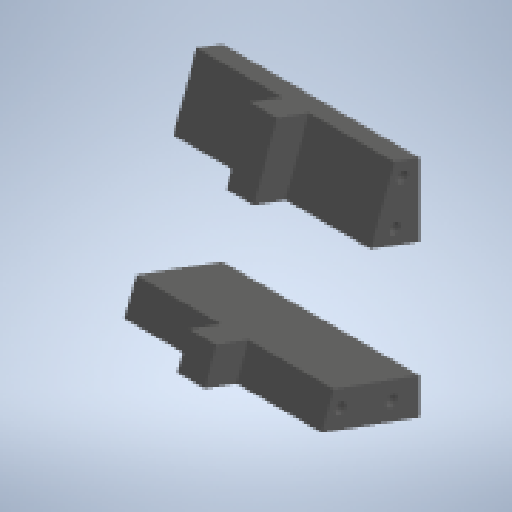
# Autodesk Inventor part: chest_cover_bace
Saved by Autodesk Inventor 2024.1 (Build 281209000, 209)
## iProperties
Created: 2024-02-14
Part Number: chest_cover_bace
Material: 一般
Document SubType Name: Modeling
Designer: hibik
Density: 1 g/cm^3
Appearance: 既定
Author: hibik
Autodesk Inventor part; units mm, degrees
ref_plane "YZ Plane" through (0, 0, 0) normal (1, 0, 0) x (0, 1, 0)
ref_plane "XZ Plane" through (0, 0, 0) normal (0, 1, 0) x (-1, 0, 0)
ref_plane "XY Plane" through (0, 0, 0) normal (0, 0, 1) x (1, 0, 0)
sketch "スケッチ1" plane through (0, 0, 0) normal (1, 0, 0) x (0, 1, 0)
  line L0 (0, 0) -> (33, 0)
  line L1 (33, 0) -> (3.8603, 10.606)
  line L2 (3.8603, 10.606) -> (0, 0)
  line L3 (33, 0) -> (3.8603, 10.606)
  line L4 (3.8603, 10.606) -> (5.2283, 14.3648)
  line L5 (5.2283, 14.3648) -> (34.3681, 3.7588)
  line L6 (34.3681, 3.7588) -> (33, 0)
  dimension "d0" = 33
  dimension "d1" = 20
  dimension "d2" = 4
  constraints: 14 end point, 3 equal length, 2 perpendicular, 1 horizontal
  measures "d0" distance of L0.start L0.end
  measures "d1" angle of L0 L1
  measures "d2" distance between parallel lines of L5 L1
extrude "押し出し1" add sketch "スケッチ1" along normal blind 16.5
sketch "スケッチ2" plane through (0, 5.2283, 14.3648) normal (0, 0.3420201, 0.9396926) x (1, 0, 0)
  line L0 (0, 31.0099) -> (16.5, 31.0099) projected
  line L1 (16.5, 31.0099) -> (16.5, 0) projected
  line L2 (12.5, 31.0099) -> (16.5, 31.0099)
  line L3 (16.5, 31.0099) -> (16.5, 0)
  line L4 (16.5, 0) -> (12.5, 0)
  line L5 (12.5, 0) -> (12.5, 31.0099)
  point P0 (0, 0)
  dimension "d5" = 4
  constraints: 8 end point, 2 parallel, 1 horizontal, 1 perpendicular, 1 point on line
  measures "d5" distance between parallel lines of L1 L5
extrude "押し出し2" add sketch "スケッチ2" along normal blind 5
extrude "押し出し3" add sketch "スケッチ1" along normal blind 29
sketch "スケッチ3" plane through (0, 0, 0) normal (-1, 0, 0) x (0, 0, 1)
  line L0 (3.7588, 34.3681) -> (14.3648, 5.2283) projected
  line L1 (7.179, 24.9712) -> (12.6547, 9.9268)
  line L2 (12.6547, 9.9268) -> (0, 5.3209)
  line L3 (0, 5.3209) -> (-5.4757, 20.3652)
  line L4 (-5.4757, 20.3652) -> (7.179, 24.9712)
  line L5 (0, 0) -> (0, 33) projected
  line L6 (0, 33) -> (3.7588, 34.3681) projected
  line L7 (14.3648, 5.2283) -> (0, 0) projected
  circle A0 centre (11.6303, 6.8935) radius 0.8
  circle A1 centre (4.1128, 4.1574) radius 0.8
  circle A2 centre (2.5634, 31.8047) radius 0.8
  circle A3 centre (3.6759, 25.8245) radius 0.8
  line L8 (7.179, 24.9712) -> (12.6547, 9.9268)
  line L9 (12.6547, 9.9268) -> (17.3531, 11.6369)
  line L10 (17.3531, 11.6369) -> (11.8774, 26.6813)
  line L11 (11.8774, 26.6813) -> (7.179, 24.9712)
  point P0 (0, 22.3582)
  dimension "d13" = 10
  dimension "d14" = 5
  dimension "d15" = 1.6
  dimension "d16" = 1.6
  dimension "d17" = 1.6
  dimension "d18" = 1.6
  dimension "d19" = 2.5
  dimension "d20" = 2.5
  dimension "d21" = 2
  dimension "d22" = 3
  dimension "d23" = 2
  dimension "d24" = 2
  dimension "d25" = 2
  dimension "d26" = 10
  constraints: 16 end point, 4 centre point, 4 parallel, 3 point on line, 2 perpendicular, 1 collinear
  measures "d13" distance between parallel lines of L6 L4
  measures "d14" distance between parallel lines of L7 L2
  measures "d15" diameter of A0
  measures "d16" diameter of A1
  measures "d17" diameter of A2
  measures "d18" diameter of A3
  measures "d19" distance from line of L7 A0.centre
  measures "d20" distance from line of L7 A1.centre
  measures "d21" distance from line of L0 A2.centre
  measures "d22" distance from line of L0 A3.centre
  measures "d23" distance from line of L4 A3.centre
  measures "d24" distance from line of L6 A2.centre
  measures "d25" distance from line of L0 A0.centre
  measures "d26" distance from line of L0 A1.centre
extrude "押し出し4" cut sketch "スケッチ3" against normal through all contours L11 L10 L9 L0 | L0 L2 L5 L4 | L5 L3 L4 | A0 | A1 | A2 | A3
equation "\"d20\" = d19"
